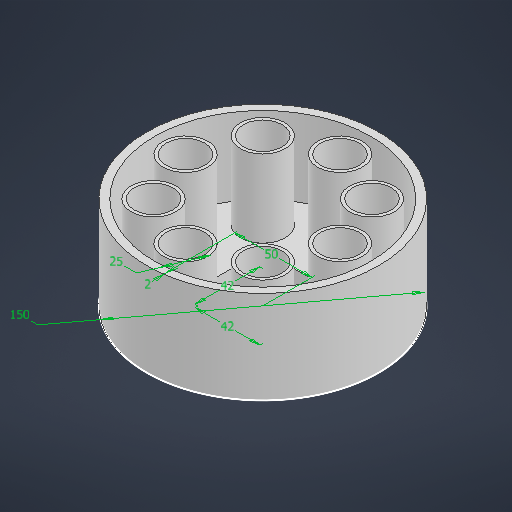
# Autodesk Inventor part: bottom
Saved by Autodesk Inventor 2025.1 (Build 291241000, 241)
## iProperties
Created: 2025-02-19
Part Number: bottom
Material: Generic
Document SubType Name: Modeling
Designer: jerem
Density: 1 g/cm^3
Appearance: Default
Author: jerem
Autodesk Inventor part; units mm, degrees
ref_plane "YZ Plane" through (0, 0, 0) normal (1, 0, 0) x (0, 1, 0)
ref_plane "XZ Plane" through (0, 0, 0) normal (0, 1, 0) x (-1, 0, 0)
ref_plane "XY Plane" through (0, 0, 0) normal (0, 0, 1) x (1, 0, 0)
sketch "Sketch1" plane through (0, 0, 0) normal (0, 1, 0) x (-1, 0, 0)
  line L0 (-21, -21) -> (21, -21)
  line L1 (21, -21) -> (21, 21)
  line L2 (21, 21) -> (-21, 21)
  line L3 (-21, 21) -> (-21, -21)
  line L4 (-21, -21) -> (21, 21) construction
  line L5 (21, -21) -> (-21, 21) construction
  circle A0 centre (0, 0) radius 75
  circle A1 centre (50, 0) radius 12.5
  circle A2 centre (50, 0) radius 14.5
  line L6 (50, 0) -> (0, 0) construction
  dimension "d0" = 42
  dimension "d1" = 42
  dimension "d2" = 150
  dimension "d3" = 50
  dimension "d4" = 2
  dimension "d5" = 25
  constraints: 14 end point, 3 centre point, 2 coincident, 2 horizontal, 2 midpoint, 2 parallel, 1 perpendicular
  measures "d0" distance of L2.end L1.end
  measures "d1" distance of L1.end L0.end
  measures "d2" diameter of A0
  measures "d3" distance of point (0, 0) A1.centre
  measures "d4" radial gap between concentric circles of A1 A2
  measures "d5" diameter of A1
extrude "Extrusion1" add sketch "Sketch1" along normal blind 10 contours A0 | A1 | A2
extrude "Extrusion2" add sketch "Sketch1" along normal blind 50 from surface at 10 contours A2
sketch "Sketch2" plane through (0, 10, 0) normal (0, 1, 0) x (1, 0, 0)
  circle A0 centre (-50, 0) radius 14.5 projected
  line L0 (21, 21) -> (21, -21) projected
  line L1 (21, -21) -> (-21, -21) projected
  line L2 (-21, -21) -> (-21, 21) projected
  line L3 (-21, 21) -> (21, 21) projected
  circle A1 centre (0, 0) radius 75 projected
  circle A2 centre (0, 0) radius 70
  dimension "d10" = 5
  constraints: 1 centre point
  measures "d10" radial gap between concentric circles of A1 A2
extrude "Extrusion3" add sketch "Sketch2" along normal blind 50 contours A1
pattern_circular "Circular Pattern1" count 8 over 360 about axis through (0, 0, 0) along (0, 1, 0) of "Extrusion2"
body "Solid1"
